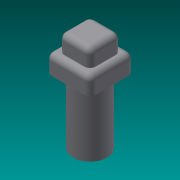
# Autodesk Inventor part: Power Switch
Saved by Autodesk Inventor 2015 (Build 190159000, 159)
## iProperties
Created: 2015-01-31
Part Number: Power Switch
Material: Generic
Document SubType Name: Modeling
Designer: Sawaiz Syed
Density: 1 g/cm^3
Appearance: Default
Author: Sawaiz Syed
Autodesk Inventor part; units mm, degrees
ref_plane "YZ Plane" through (0, 0, 0) normal (1, 0, 0) x (0, 1, 0)
ref_plane "XZ Plane" through (0, 0, 0) normal (0, 1, 0) x (-1, 0, 0)
ref_plane "XY Plane" through (0, 0, 0) normal (0, 0, 1) x (1, 0, 0)
sketch "Sketch1" plane through (0, 0, 0) normal (0, 0, 1) x (1, 0, 0)
  circle A0 centre (0, 0) radius 6
  dimension "d0" = 12
  constraints: 1 centre point, 1 coincident
  measures "d0" diameter of A0
extrude "Extrusion1" add sketch "Sketch1" along normal blind 22.9
sketch "Sketch2" plane through (0, 0, 22.9) normal (0, 0, 1) x (1, 0, 0)
  line L0 (-7.75, 7.75) -> (7.75, 7.75)
  line L1 (7.75, 7.75) -> (7.75, -7.75)
  line L2 (7.75, -7.75) -> (-7.75, -7.75)
  line L3 (-7.75, -7.75) -> (-7.75, 7.75)
  line L4 (-7.75, 7.75) -> (7.75, -7.75) construction
  line L5 (7.75, 7.75) -> (-7.75, -7.75) construction
  point P0 (0, 0)
  dimension "d3" = 15.5
  dimension "d4" = 15.5
  constraints: 12 end point, 2 midpoint, 2 parallel, 1 horizontal, 1 perpendicular
  measures "d3" distance of L1.end L2.end
  measures "d4" distance of L0.end L1.end
extrude "Extrusion2" add sketch "Sketch2" along normal blind 6.4
sketch "Sketch3" plane through (0, 0, 29.3) normal (0, 0, 1) x (1, 0, 0)
  line L0 (-5.5, 5.5) -> (5.5, 5.5)
  line L1 (5.5, 5.5) -> (5.5, -5.5)
  line L2 (5.5, -5.5) -> (-5.5, -5.5)
  line L3 (-5.5, -5.5) -> (-5.5, 5.5)
  line L4 (-5.5, 5.5) -> (5.5, -5.5) construction
  line L5 (5.5, 5.5) -> (-5.5, -5.5) construction
  point P0 (0, 0)
  dimension "d7" = 11
  dimension "d8" = 11
  constraints: 12 end point, 2 midpoint, 2 parallel, 1 horizontal, 1 perpendicular
  measures "d7" distance of L1.end L2.end
  measures "d8" distance of L0.end L1.end
extrude "Extrusion3" add sketch "Sketch3" along normal blind 6
fillet "Fillet1" radius 2 12 edges at (0, 5.5, 35.3) (5.5, 5.5, 32.3) (5.5, 0, 35.3) (0, -5.5, 35.3) (5.5, -5.5, 32.3) (-5.5, 0, 35.3) (-5.5, 5.5, 32.3) (-5.5, -5.5, 32.3) (-7.75, 0, 29.3) (0, -7.75, 29.3) (7.75, 0, 29.3) (0, 7.75, 29.3)
fillet "Fillet2" radius 2 8 edges at (7.1642, -7.1642, 28.7142) (7.75, -7.75, 25.1) (-7.1642, -7.1642, 28.7142) (-7.75, -7.75, 25.1) (7.1642, 7.1642, 28.7142) (7.75, 7.75, 25.1) (-7.1642, 7.1642, 28.7142) (-7.75, 7.75, 25.1)
body "Solid1"
